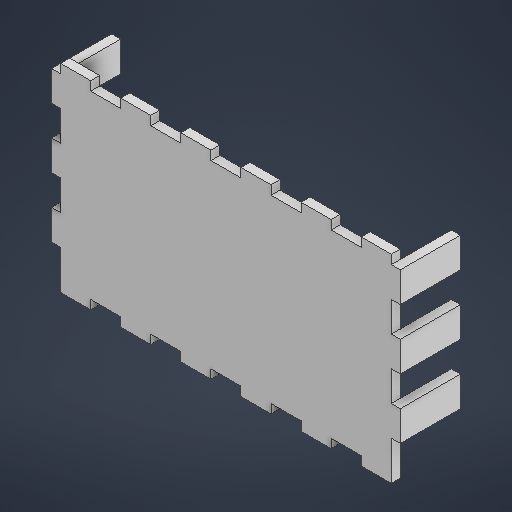
# Autodesk Inventor part: portada
Saved by Autodesk Inventor 2026 (Build 300175000, 175)
## iProperties
Created: 2026-04-21
Part Number: portada
Material: Generic
Document SubType Name: Modeling
Designer: juana
Density: 1 g/cm^3
Appearance: Default
Author: juana
Autodesk Inventor part; units mm, degrees
ref_plane "YZ Plane" through (0, 0, 0) normal (1, 0, 0) x (0, 1, 0)
ref_plane "XZ Plane" through (0, 0, 0) normal (0, 1, 0) x (-1, 0, 0)
ref_plane "XY Plane" through (0, 0, 0) normal (0, 0, 1) x (1, 0, 0)
sketch "Sketch1" plane through (0, 0, 0) normal (0, 0, 1) x (1, 0, 0)
  line L0 (0, 0) -> (110, 0)
  line L1 (110, 0) -> (110, 60)
  line L2 (110, 60) -> (0, 60)
  line L3 (0, 60) -> (0, 0)
  dimension "d0" = 60
  dimension "d1" = 110
  constraints: 8 end point, 2 parallel, 1 horizontal, 1 perpendicular
  measures "d0" distance of L0.end L1.end
  measures "d1" distance of L1.end L2.end
extrude "Extrusion1" add sketch "Sketch1" along normal blind 3
sketch "Sketch2" plane through (0, 0, 3) normal (0, 0, 1) x (1, 0, 0)
  line L0 (0, 0) -> (110, 0) projected
  line L1 (0, 0) -> (10, 0)
  line L2 (10, 0) -> (10, -3)
  line L3 (10, -3) -> (0, -3)
  line L4 (0, -3) -> (0, 0)
  line L5 (20, 0) -> (30, 0)
  line L6 (30, 0) -> (30, -3)
  line L7 (30, -3) -> (20, -3)
  line L8 (20, -3) -> (20, 0)
  line L9 (40, 0) -> (50, 0)
  line L10 (50, 0) -> (50, -3)
  line L11 (50, -3) -> (40, -3)
  line L12 (40, -3) -> (40, 0)
  line L13 (60, 0) -> (70, 0)
  line L14 (70, 0) -> (70, -3)
  line L15 (70, -3) -> (60, -3)
  line L16 (60, -3) -> (60, 0)
  line L17 (80, 0) -> (90, 0)
  line L18 (90, 0) -> (90, -3)
  line L19 (90, -3) -> (80, -3)
  line L20 (80, -3) -> (80, 0)
  line L21 (100, 0) -> (110, 0)
  line L22 (110, 0) -> (110, -3)
  line L23 (110, -3) -> (100, -3)
  line L24 (100, -3) -> (100, 0)
  line L25 (0, 60) -> (0, 0) construction
  line L26 (0, 63) -> (10, 63)
  line L27 (10, 63) -> (10, 60)
  line L28 (10, 60) -> (0, 60)
  line L29 (0, 60) -> (0, 63)
  line L30 (20, 63) -> (30, 63)
  line L31 (30, 63) -> (30, 60)
  line L32 (30, 60) -> (20, 60)
  line L33 (20, 60) -> (20, 63)
  line L34 (40, 63) -> (50, 63)
  line L35 (50, 63) -> (50, 60)
  line L36 (50, 60) -> (40, 60)
  line L37 (40, 60) -> (40, 63)
  line L38 (60, 63) -> (70, 63)
  line L39 (70, 63) -> (70, 60)
  line L40 (70, 60) -> (60, 60)
  line L41 (60, 60) -> (60, 63)
  line L42 (80, 63) -> (90, 63)
  line L43 (90, 63) -> (90, 60)
  line L44 (90, 60) -> (80, 60)
  line L45 (80, 60) -> (80, 63)
  line L46 (100, 63) -> (110, 63)
  line L47 (110, 63) -> (110, 60)
  line L48 (110, 60) -> (100, 60)
  line L49 (100, 60) -> (100, 63)
  dimension "d4" = 10
  dimension "d5" = 3
  dimension "d8" = 20
  dimension "d11" = 63
  constraints: 96 end point, 2 horizontal, 2 parallel, 1 perpendicular, 1 vertical, 88 other
  measures "d4" distance of L2.end L3.end
  measures "d5" distance of L3.end L0.start
  measures "d8" distance of L2.end L6.end
  measures "d11" distance of L2.end L27.end
extrude "Extrusion2" add sketch "Sketch2" against normal blind 3
sketch "Sketch3" plane through (0, 0, 3) normal (0, 0, 1) x (1, 0, 0)
  line L0 (-3, 20) -> (0, 20)
  line L1 (0, 20) -> (0, 10)
  line L2 (0, 10) -> (-3, 10)
  line L3 (-3, 10) -> (-3, 20)
  line L4 (0, 63) -> (0, -3) construction
  line L5 (10, 0) -> (20, 0) construction
  line L6 (-3, 40) -> (0, 40)
  line L7 (0, 40) -> (0, 30)
  line L8 (0, 30) -> (-3, 30)
  line L9 (-3, 30) -> (-3, 40)
  line L10 (-3, 60) -> (0, 60)
  line L11 (0, 60) -> (0, 50)
  line L12 (0, 50) -> (-3, 50)
  line L13 (-3, 50) -> (-3, 60)
  line L14 (110, 20) -> (113, 20)
  line L15 (113, 20) -> (113, 10)
  line L16 (113, 10) -> (110, 10)
  line L17 (110, 10) -> (110, 20)
  line L18 (110, 40) -> (113, 40)
  line L19 (113, 40) -> (113, 30)
  line L20 (113, 30) -> (110, 30)
  line L21 (110, 30) -> (110, 40)
  line L22 (110, 60) -> (113, 60)
  line L23 (113, 60) -> (113, 50)
  line L24 (113, 50) -> (110, 50)
  line L25 (110, 50) -> (110, 60)
  point P0 (0, 0)
  dimension "d16" = 3
  dimension "d17" = 10
  dimension "d18" = 10
  dimension "d21" = 20
  dimension "d24" = 113
  constraints: 48 end point, 2 horizontal, 2 parallel, 1 perpendicular, 1 vertical, 1 vertical alignment, 40 other
  measures "d16" distance of L0.start L0.end
  measures "d17" distance of L2.end L0.start
  measures "d18" distance from line of point (0, 0) L2
  measures "d21" distance of L0.start L6.start
  measures "d24" distance of L0.start L14.start
extrude "Extrusion3" add sketch "Sketch3" against normal blind 20
equation "\"d27\" = d21"
body "Solid1"
